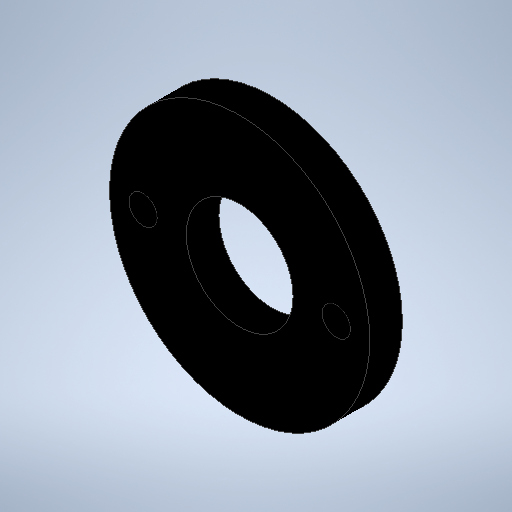
# Autodesk Inventor part: Red Pump Flange
Saved by Autodesk Inventor 2027 (Build 310192000, 192)
## iProperties
Created: 2026-09-05
Part Number: Red Pump Flange
Material: Generic
Document SubType Name: Modeling
Designer: IG2
Density: 1 g/cm^3
Appearance: Default
Author: IG2
Autodesk Inventor part; units mm, degrees
ref_plane "YZ Plane" through (0, 0, 0) normal (1, 0, 0) x (0, 1, 0)
ref_plane "XZ Plane" through (0, 0, 0) normal (0, 1, 0) x (-1, 0, 0)
ref_plane "XY Plane" through (0, 0, 0) normal (0, 0, 1) x (1, 0, 0)
sketch "Sketch1" plane through (0, 0, 0) normal (0, 0, 1) x (1, 0, 0)
  circle A0 centre (0, 0) radius 24.13
  circle A1 centre (0, 0) radius 58.7375
  circle A2 centre (43.6372, 0) radius 6.35
  line L0 (0, 24.13) -> (0, 58.7375)
  circle A3 centre (-43.6372, 0) radius 6.35
  dimension "d0" = 48.26
  dimension "d1" = 117.475
  dimension "d4" = 12.7
  dimension "d5" = 43.6372
  constraints: 2 centre point, 2 coincident, 2 end point, 2 vertical alignment, 1 symmetric about line, 1 vertical, 5 other
  measures "d4" diameter of A2
  measures "d5" distance of A2.centre point (0, 0)
extrude "Extrusion1" add sketch "Sketch1" against normal blind 14.732 contours A1 | A2 | A3
extrude "Extrusion2" cut sketch "Sketch1" against normal through all contours A2 | A3
body "Solid1"
